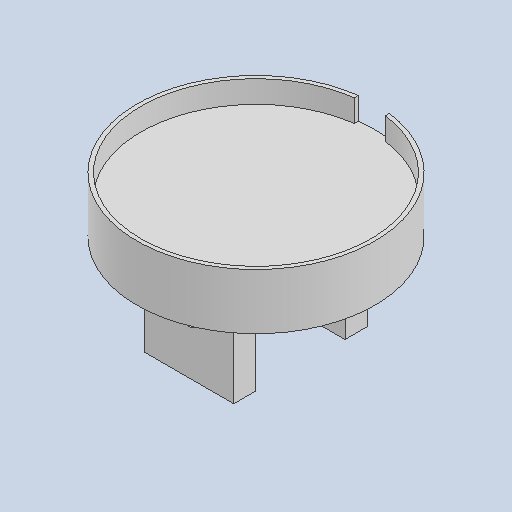
# Autodesk Inventor part: lidar_case
Saved by Autodesk Inventor 2025.2 (Build 292293000, 293)
## iProperties
Created: 2024-02-08
Part Number: lidar_case
Material: 일반
Document SubType Name: Modeling
Designer: ps737
Density: 1 g/cm^3
Appearance: 기본값
Author: ps737
Autodesk Inventor part; units mm, degrees
ref_plane "YZ Plane" through (0, 0, 0) normal (1, 0, 0) x (0, 1, 0)
ref_plane "XZ Plane" through (0, 0, 0) normal (0, 1, 0) x (-1, 0, 0)
ref_plane "XY Plane" through (0, 0, 0) normal (0, 0, 1) x (1, 0, 0)
sketch "스케치1" plane through (0, 0, 0) normal (0, 1, 0) x (-1, 0, 0)
  circle A0 centre (0, 0) radius 51.635
  circle A1 centre (0, 0) radius 53.4089
  dimension "d0" = 103.27
  constraints: 2 centre point, 2 coincident
  measures "d0" diameter of A0
extrude "돌출1" add sketch "스케치1" along normal blind 25
extrude "돌출2" add sketch "스케치1" along normal blind 15 contours A0
sketch "스케치2" plane through (0, 25, 0) normal (0, 1, 0) x (1, 0, 0)
  line L0 (-7, 38.0484) -> (-7, 59.2742)
  line L1 (7, 38.0484) -> (7, 59.2742)
  circle A0 centre (0, 0) radius 53.4089 projected
  circle A1 centre (0, 0) radius 51.635 projected
  point P0 (-7, 51.1583)
  point P1 (7, 51.1583)
  point P2 (7, 52.9482)
  point P3 (-7, 52.9482)
  dimension "d5" = 14
  dimension "d6" = 7
  constraints: 4 end point, 2 vertical
  measures "d5" distance between parallel lines of L1 L0
  measures "d6" distance from line of point (0, 0) L0
extrude "돌출3" cut sketch "스케치2" against normal blind 10 contours L0 A0 L1 A1 picked at (5.4466, 51.8962)
sketch "스케치5" plane through (0, 0, 0) normal (0, -1, 0) x (1, 0, 0)
  circle A0 centre (0, 0) radius 53.4089 projected
  line L0 (0, 53.4089) -> (0, -53.4089) construction
  line L1 (-53.4089, 0) -> (53.4089, 0) construction
  line L2 (-49.5229, 20) -> (49.5229, 20) construction
  line L3 (49.5229, 20) -> (49.5229, -20) construction
  line L4 (49.5229, -20) -> (-49.5229, -20) construction
  line L5 (-49.5229, -20) -> (-49.5229, 20) construction
  line L6 (-20, 20) -> (20, 20)
  line L7 (20, 20) -> (20, 30)
  line L8 (20, 30) -> (-20, 30)
  line L9 (-20, 30) -> (-20, 20)
  line L10 (20, -20) -> (20, -30)
  line L11 (20, -30) -> (-20, -30)
  line L12 (-20, -30) -> (-20, -20)
  line L13 (-20, -20) -> (20, -20)
  point P0 (0, 30)
  dimension "d19" = 40
  dimension "d20" = 20
  dimension "d21" = 40
  dimension "d22" = 10
  constraints: 28 end point, 6 point on circle, 4 parallel, 4 symmetric about line, 3 horizontal, 3 midpoint, 3 perpendicular, 2 point on line, 1 vertical
  measures "d19" distance of L2.end L3.end
  measures "d20" distance between parallel lines of L1 L2
  measures "d21" distance of L8.end L7.end
  measures "d22" distance of L7.end L6.end
extrude "돌출6" add sketch "스케치5" along normal blind 40 contours L9 L8 L7 L6 | L10 L11 L12 L13
sketch "스케치6" plane through (-20, 0, 30) normal (0, 0, 1) x (1, 0, 0)
  line L0 (0, 0) -> (40, 0) projected
  line L1 (0, 0) -> (0, -40) projected
  line L2 (40, -40) -> (0, -40) projected
  line L3 (40, 0) -> (40, -40) projected
  circle A0 centre (20, -16.074) radius 4
  point P0 (20, 0)
  dimension "d25" = 8
  dimension "d26" = 16.074
  dimension "d27" = 20
  constraints: 1 centre point
  measures "d25" diameter of A0
  measures "d26" distance from line of L0 A0.centre
  measures "d27" distance from line of L1 A0.centre
extrude "돌출7" cut sketch "스케치6" against normal blind 69.75 contours A0
